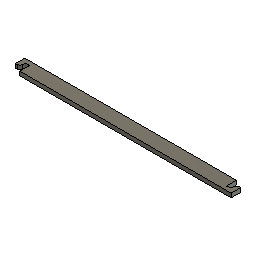
SyncLedStripBase (Autodesk Fusion 360 design; units mm, degrees)
Autodesk Fusion 360 part; units mm, degrees
sketch "Sketch1" plane through (0, 0, 0) normal (0, 1, 0) x (1, 0, 0)
  line L0 (-160, 0) -> (-160, -6.8)
  line L1 (0, -10) -> (-3, -10)
  line L2 (-1, -3) -> (0, -3)
  line L3 (0, -3) -> (0, -10)
  arc A0 (-1, -3) -> (-2.9926, -5.1721) centre (-1, -5) ccw
  line L4 (-6.1852, 0) -> (-6.1852, -7)
  line L5 (-6.1852, -7) -> (-4.9852, -7)
  arc A1 (-4.9852, -7) -> (-2.9852, -5) centre (-4.9852, -5) ccw
  line L6 (0, -10) -> (0, -3)
  line L7 (-2.9852, -5) -> (-3, -5)
  line L8 (-158.8202, -6.8) -> (-160, -6.8)
  arc A2 (-158.8202, -6.8) -> (-156.8276, -4.6279) centre (-158.8202, -4.8) ccw
  arc A3 (-154.8351, -2.8) -> (-156.8351, -4.8) centre (-154.8351, -4.8) ccw
  line L9 (-153.6351, -2.8) -> (-154.8351, -2.8)
  line L10 (-153.6351, -10) -> (-153.6351, -2.8)
  line L11 (-153.6351, -10) -> (0, -10)
  line L12 (-6.1852, 0) -> (-160, 0)
  point P0 (-2.9852, -7)
  dimension "d1" = 160
  dimension "d2" = 10
  dimension "d3" = 3
  dimension "d4" = 7
  dimension "d5" = 2
  dimension "d8" = 2
  dimension "d9" = 2
  dimension "d10" = 2
  constraint vertical L0
  constraint horizontal L1
  constraint horizontal L2
  constraint vertical L3
  constraint tangent L2 A0
  constraint vertical L4
  constraint horizontal L5
  constraint coincident P0 L5
  constraint tangent L5 A1
  constraint horizontal L7
  constraint tangent L8 A2
  constraint tangent A3 L9
  constraint horizontal L11
  constraint horizontal L12
  constraint coincident A1 A0.end
  constraint coincident L7.end A0
  constraint coincident A3 A2.end
  measures "d1" distance of origin L0.start
  measures "d2" distance of origin L1.start
  measures "d3" distance of L1.start L1.end
  measures "d4" distance of L1.start L2.end
  measures "d5" radius of A0
  measures "d8" radius of A1
  measures "d9" radius of A2
  measures "d10" radius of A3
extrude "Extrude1" add sketch "Sketch1" along normal blind 3 contours L0 L1 L2 L3 A0 L4 L5 A1 L6 L7 L8 A2 A3 L9 L10 L11 L12
